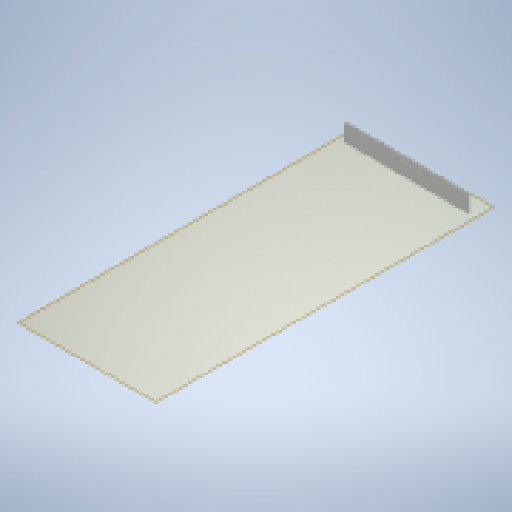
# Autodesk Inventor part: SeilatrappeHalter
Saved by Autodesk Inventor 2025 (Build 290162010, 162A)
## iProperties
Created: 2024-11-19
Part Number: SeilatrappeHalter
Material: Generisch
Document SubType Name: Modeling
Designer: Admin
Density: 1 g/cm^3
Appearance: Vorgabe
Author: Admin
Autodesk Inventor part; units mm, degrees
ref_plane "YZ Plane" through (0, 0, 0) normal (1, 0, 0) x (0, 1, 0)
ref_plane "XZ Plane" through (0, 0, 0) normal (0, 1, 0) x (-1, 0, 0)
ref_plane "XY Plane" through (0, 0, 0) normal (0, 0, 1) x (1, 0, 0)
ref_plane "Arbeitsebene1" through (0, 0, 0) normal (0, 0, 1) x (1, 0, 0)
sketch "Skizze1" plane through (0, 0, 0) normal (0, 0, 1) x (1, 0, 0)
  line L0 (0, 490) -> (200, 490) projected
  line L1 (0, 490) -> (200, 490)
  line L2 (200, 490) -> (200, 485)
  line L3 (200, 485) -> (0, 485)
  line L4 (0, 485) -> (0, 490)
  point P0 (0, 0)
  dimension "d0" = 5
  constraints: 8 end point, 2 parallel, 1 horizontal, 1 perpendicular, 1 point on line
  measures "d0" distance of L1.end L2.end
extrude "Extrusion1" add sketch "Skizze1" along normal blind 25
sketch "Skizze2" plane through (0, 485, 0) normal (0, -1, 0) x (1, 0, 0)
  arc A0 (77.7509, 20) -> (81.7509, 20) centre (79.7509, 20) ccw
  arc A1 (117.7509, 20) -> (121.7509, 20) centre (119.7509, 20) ccw
  arc A2 (104.6667, 20) -> (108.6667, 20) centre (106.6667, 20) ccw
  arc A3 (91.3333, 20) -> (95.3333, 20) centre (93.3333, 20) ccw
  point P0 (0, 0)
  constraints: 8 point on circle, 4 centre point, 2 coincident, 16 other
hole "Bohrung1" at (119.7509, 485, 20) at (106.6667, 485, 20) at (93.3333, 485, 20) at (79.7509, 485, 20) direction (0, 1, 0) diameter 3 end through all
